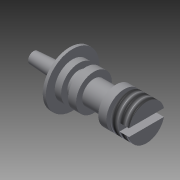
# Autodesk Inventor part: Carburetor
Saved by Autodesk Inventor 2015 (Build 190159000, 159)
## iProperties
Created: 2016-02-14
Part Number: Carburetor
Material: Generic
Document SubType Name: Modeling
Designer: Owner
Density: 1 g/cm^3
Appearance: Default
Mass: 0.280386 g
Surface Area: 5.32083 cm^2
Volume: 0.280386 cm^3
Author: Owner
Autodesk Inventor part; units mm, degrees
ref_plane "YZ Plane" through (0, 0, 0) normal (1, 0, 0) x (0, 1, 0)
ref_plane "XZ Plane" through (0, 0, 0) normal (0, 1, 0) x (-1, 0, 0)
ref_plane "XY Plane" through (0, 0, 0) normal (0, 0, 1) x (1, 0, 0)
sketch "Sketch1" plane through (0, 0, 0) normal (0, 0, 1) x (1, 0, 0)
  line L0 (0, 0) -> (18.7452, 0)
  line L1 (18.7452, 0) -> (18.7452, 2.9718)
  line L2 (18.7452, 2.9718) -> (15.6972, 2.9718)
  line L3 (15.6972, 2.9718) -> (15.6972, 1.9558)
  line L4 (15.6972, 1.9558) -> (15.0622, 1.9558)
  line L5 (15.0622, 1.9558) -> (15.0622, 2.9718)
  line L6 (15.0622, 2.9718) -> (13.716, 2.9718)
  line L7 (13.716, 2.9718) -> (13.716, 1.9558)
  line L8 (13.716, 1.9558) -> (10.033, 1.9558)
  line L9 (10.033, 1.9558) -> (10.033, 2.9718)
  line L10 (10.033, 2.9718) -> (8.6868, 2.9718)
  line L11 (8.6868, 2.9718) -> (8.6868, 1.9558)
  line L12 (8.6868, 1.9558) -> (7.5438, 1.9558)
  line L13 (7.5438, 1.9558) -> (7.5438, 2.9718)
  line L14 (7.5438, 2.9718) -> (6.477, 2.9718)
  line L15 (6.477, 2.9718) -> (6.477, 4.445)
  line L16 (6.477, 4.445) -> (5.969, 4.445)
  line L17 (5.969, 4.445) -> (5.969, 1.2785)
  line L18 (0, 0) -> (0, 0.9144)
  line L19 (0, 0.9144) -> (5.969, 1.2785)
  dimension "d0" = 18.7452
  dimension "d1" = 2.9718
  dimension "d2" = 3.048
  dimension "d3" = 1.016
  dimension "d4" = 0.635
  dimension "d5" = 1.3462
  dimension "d6" = 3.683
  dimension "d7" = 1.3462
  dimension "d8" = 1.143
  dimension "d9" = 1.0668
  dimension "d10" = 1.4732
  dimension "d11" = 0.508
  dimension "d12" = 0.9144
  constraints: 40 end point, 9 vertical, 8 horizontal, 2 perpendicular
  measures "d0" distance of L0.start L0.end
  measures "d1" distance of L0.end L1.end
  measures "d2" distance of L1.end L2.end
  measures "d3" distance of L2.end L3.end
  measures "d4" distance of L3.end L4.end
  measures "d5" distance of L5.end L6.end
  measures "d6" distance of L7.end L8.end
  measures "d7" distance of L9.end L10.end
  measures "d8" distance of L11.end L12.end
  measures "d9" distance of L13.end L14.end
  measures "d10" distance of L14.end L15.end
  measures "d11" distance of L15.end L16.end
  measures "d12" distance of L0.start L18.end
revolve "Revolution1" add sketch "Sketch1" angle 360 about axis through (0, 0, 0) along (1, 0, 0)
hole "Hole1" at (0, 0, 0) direction (1, 0, 0) diameter 1.27 depth 12.319 tip angle 118
thread "Thread1" size "1/4-20 UNC" class "2A" standard "ANSI Unified Screw Threads" full length
sketch "Sketch2" plane through (18.7452, 0, 0) normal (1, 0, 0) x (0, 0, -1)
  circle A0 centre (0, 0) radius 2.9718 projected
  line L0 (0, 0) -> (0, 0.635)
  line L1 (0, 0.635) -> (-2.9972, 0.635)
  line L2 (-2.9972, 0.635) -> (2.9718, 0.635)
  line L3 (2.9718, 0.635) -> (2.9718, -0.635)
  line L4 (2.9718, -0.635) -> (-2.9972, -0.635)
  line L5 (-2.9972, -0.635) -> (-2.9972, 0.635)
  dimension "d25" = 0.635
  dimension "d26" = 2.9972
  dimension "d27" = 5.969
  dimension "d28" = 1.27
  constraints: 12 end point, 2 horizontal, 2 parallel, 1 perpendicular, 1 vertical
  measures "d25" distance of L0.start L0.end
  measures "d26" distance of L0.end L1.end
  measures "d27" distance of L3.end L4.end
  measures "d28" distance of L2.end L3.end
extrude "Extrusion1" cut sketch "Sketch2" against normal blind 1.5875 contours A0 L4 L1 L2 | L3 L4 A0 | A0 L2 L3 | A0 L4 L5 L1
sketch "Sketch3" plane through (0, 0, 0) normal (0, 0, 1) x (1, 0, 0)
  line L0 (0, 0) -> (12.319, 0)
  dimension "d31" = 12.319
  constraints: 2 end point, 1 horizontal
  measures "d31" distance of L0.start L0.end
hole "Hole2" at (12.319, 0, 0) direction (0, 0, -1) diameter 0.7874 end through all
body "Solid1"
